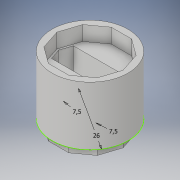
# Autodesk Inventor part: Probe P2
Saved by Autodesk Inventor 2019 (Build 230136000, 136)
## iProperties
Created: 2019-07-29
Part Number: Probe P2
Material: Generic
Document SubType Name: Modeling
Designer: azriel
Density: 1 g/cm^3
Appearance: Default
Author: azriel
Autodesk Inventor part; units mm, degrees
ref_plane "YZ Plane" through (0, 0, 0) normal (1, 0, 0) x (0, 1, 0)
ref_plane "XZ Plane" through (0, 0, 0) normal (0, 1, 0) x (-1, 0, 0)
ref_plane "XY Plane" through (0, 0, 0) normal (0, 0, 1) x (1, 0, 0)
sketch "Sketch1" plane through (0, 0, 0) normal (0, 1, 0) x (-1, 0, 0)
  circle A0 centre (0, 0) radius 13
  line L0 (-10.6616, 0) -> (-8.6254, 6.2667)
  line L1 (-8.6254, 6.2667) -> (-3.2946, 10.1398)
  line L2 (-3.2946, 10.1398) -> (3.2946, 10.1398)
  line L3 (3.2946, 10.1398) -> (8.6254, 6.2667)
  line L4 (8.6254, 6.2667) -> (10.6616, 0)
  line L5 (10.6616, 0) -> (8.6254, -6.2667)
  line L6 (8.6254, -6.2667) -> (3.2946, -10.1398)
  line L7 (3.2946, -10.1398) -> (-3.2946, -10.1398)
  line L8 (-3.2946, -10.1398) -> (-8.6254, -6.2667)
  line L9 (-8.6254, -6.2667) -> (-10.6616, 0)
  line L10 (-11.3, 0) -> (-9.1419, 6.642)
  line L11 (-9.1419, 6.642) -> (-3.4919, 10.7469)
  line L12 (-3.4919, 10.7469) -> (3.4919, 10.7469)
  line L13 (3.4919, 10.7469) -> (9.1419, 6.642)
  line L14 (9.1419, 6.642) -> (11.3, 0)
  line L15 (11.3, 0) -> (9.1419, -6.642)
  line L16 (9.1419, -6.642) -> (3.4919, -10.7469)
  line L17 (3.4919, -10.7469) -> (-3.4919, -10.7469)
  line L18 (-3.4919, -10.7469) -> (-9.1419, -6.642)
  line L19 (-9.1419, -6.642) -> (-11.3, 0)
  circle A1 centre (-6, 0) radius 3.75
  circle A2 centre (6, 0) radius 3.75
  line L20 (9.4432, -3.75) -> (-9.4432, -3.75)
  line L21 (-9.4432, 3.75) -> (9.4432, 3.75)
  dimension "d0" = 26
  dimension "d8" = 7.5
  dimension "d9" = 7.5
  constraints: 44 end point, 4 point on line, 3 centre point, 2 coincident, 1 horizontal, 1 parallel, 21 other
  measures "d0" diameter of A0
  measures "d8" diameter of A1
  measures "d9" diameter of A2
extrude "Extrusion1" add sketch "Sketch1" against normal blind 3 contours L10 L11 L12 L13 L14 L15 L16 L17 L18 L19
extrude "Extrusion2" add sketch "Sketch1" along normal blind 20 contours A0
extrude "Extrusion3" add sketch "Sketch1" along normal blind 15 contours L0 L1 L2 L3 L4 L21 | L20 L5 L6 L7 L8 L9 | L10 L11 L12 L13 L14 L15 L16 L17 L18 L19
body "Solid1"
